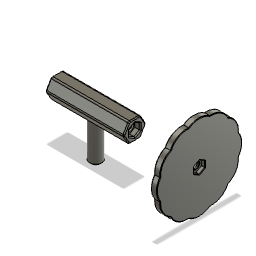
Interferometry Fine Adjust v5 (Autodesk Fusion 360 design; units mm, degrees)
Autodesk Fusion 360 part; units mm, degrees
note: some values were not read from the file. Chosen so that the rebuilt part matches the saved one: where a step starts; where a step ends.
sketch "Post" plane through (0, 0, 0) normal (0, 1, 0) x (1, 0, 0) in component "Fine Adjust Mount"
  circle A0 centre (0, 0) radius 6.25
  dimension "d1" = 12.5
  constraint coincident A0.centre origin
  measures "d1" diameter of A0
sketch "Shaft" plane through (0, 0, 0) normal (1, 0, 0) x (0, 0, -1) in component "Fine Adjust Mount"
  line L0 (0, 0) -> (5.5, 0) construction
  line L1 (0, 0) -> (0, -10) construction
  line L2 (5.5, 3.1754) -> (0, 6.3509)
  line L3 (0, 6.3509) -> (-5.5, 3.1754)
  line L4 (-5.5, 3.1754) -> (-5.5, -3.1754)
  line L5 (-5.5, -3.1754) -> (0, -6.3509)
  line L6 (0, -6.3509) -> (5.5, -3.1754)
  line L7 (5.5, -3.1754) -> (5.5, 3.1754)
  line L8 (5.7735, -10) -> (11.547, 0)
  line L9 (11.547, 0) -> (5.7735, 10)
  line L10 (5.7735, 10) -> (-5.7735, 10)
  line L11 (-5.7735, 10) -> (-11.547, 0)
  line L12 (-11.547, 0) -> (-5.7735, -10)
  line L13 (-5.7735, -10) -> (5.7735, -10)
  circle A0 centre (0, 0) radius 3.5
  dimension "d2" = 5.5
  dimension "d3" = 10
  dimension "d4" = 5.5
  dimension "d5" = 10
  dimension "d15" = 7
  constraint coincident L0.start L1.start
  constraint horizontal L0
  constraint perpendicular L0 L1
  constraint perpendicular L0 L7
  constraint perpendicular L1 L13
  measures "d2" distance of L0.start L0.end
  measures "d3" distance of L0.start L1.end
  measures "d4" distance of L0.start L7
  measures "d5" distance of L0.start L13
  measures "d15" diameter of A0
sketch "Disk" plane through (0, 0, 0) normal (1, 0, 0) x (0, 0, -1) in component "Fine Adjust Mount"
  line L0 (0, 0) -> (43.5, 0) construction
  line L1 (0, 0) -> (40.0859, 10.741) construction
  line L2 (0, 0) -> (42.5, 0) construction
  line L3 (0, 0) -> (40.0859, -10.741) construction
  line L4 (0, 0) -> (42.5, 0) construction
  arc A0 (40.0859, -10.741) -> (40.0859, 10.741) centre (24.8969, 0) ccw
  arc A1 (40.0859, 10.741) -> (29.3449, 29.3449) centre (21.5614, 12.4485) ccw
  arc A2 (29.3449, 29.3449) -> (10.741, 40.0859) centre (12.4485, 21.5614) ccw
  arc A3 (10.741, 40.0859) -> (-10.741, 40.0859) centre (0, 24.8969) ccw
  arc A4 (-10.741, 40.0859) -> (-29.3449, 29.3449) centre (-12.4485, 21.5614) ccw
  arc A5 (-29.3449, 29.3449) -> (-40.0859, 10.741) centre (-21.5614, 12.4485) ccw
  arc A6 (-40.0859, 10.741) -> (-40.0859, -10.741) centre (-24.8969, 0) ccw
  arc A7 (-40.0859, -10.741) -> (-29.3449, -29.3449) centre (-21.5614, -12.4485) ccw
  arc A8 (-29.3449, -29.3449) -> (-10.741, -40.0859) centre (-12.4485, -21.5614) ccw
  arc A9 (-10.741, -40.0859) -> (10.741, -40.0859) centre (0, -24.8969) ccw
  arc A10 (10.741, -40.0859) -> (29.3449, -29.3449) centre (12.4485, -21.5614) ccw
  arc A11 (29.3449, -29.3449) -> (40.0859, -10.741) centre (21.5614, -12.4485) ccw
  line L5 (5.5, 3.1754) -> (0, 6.3509)
  line L6 (0, 6.3509) -> (-5.5, 3.1754)
  line L7 (-5.5, 3.1754) -> (-5.5, -3.1754)
  line L8 (-5.5, -3.1754) -> (0, -6.3509)
  line L9 (0, -6.3509) -> (5.5, -3.1754)
  line L10 (5.5, -3.1754) -> (5.5, 3.1754)
  circle A12 centre (0, 0) radius 3.5
  dimension "d6" = 43.5
  dimension "d7" = 15
  dimension "d8" = 41.5
  dimension "d9" = 15
  dimension "d10" = 41.5
  dimension "d12" = 360
  dimension "d13" = 5.5
  dimension "d14" = 7
  constraint coincident L0.start L1.start
  constraint horizontal L0
  constraint horizontal L2
  constraint horizontal L4
  constraint coincident L0.end A0
  constraint perpendicular L4 L10
  measures "d6" distance of L0.start L0.end
  measures "d7" angle of L1 L2
  measures "d8" distance of L0.start L1.end
  measures "d9" angle of L3 L4
  measures "d10" distance of L0.start L3.end
  measures "d13" distance of L0.start L10
  measures "d14" diameter of A12
extrude "Extrude1" add sketch "Shaft" along normal mid plane 69 contours L2 L3 L4 L5 L6 L7 | L8 L9 L10 L11 L12 L13 makes body 1 in component "Fine Adjust Mount"
extrude "Extrude2" add sketch "Shaft" along normal mid plane 80 contours L8 L9 L10 L11 L12 L13 bodies 1 in component "Fine Adjust Mount"
extrude "Extrude3" add sketch "Post" along normal up to near side of body 1 and the other way blind 36 from surface at -11 bodies 1 in component "Fine Adjust Mount"
extrude "Extrude4" add sketch "Disk" along normal blind 6 separate body contours A0 A1 A2 A3 A4 A5 A6 A7 A8 A9 A10 A11 | L5 L6 L7 L8 L9 L10 makes body 2 in component "Fine Adjust Mount"
extrude "Extrude5" cut sketch "Disk" against normal blind 3.6667 from surface at 6 contours L5 L6 L7 L8 L9 L10 bodies 2 in component "Fine Adjust Mount"
move_body "Move1" bodies 2 to x (1, 0, 0) y (0, 1, 0) z (0, 0, 1) at (100, 0, 0) in component "Fine Adjust Mount"
fillet "Fillet2" radius 2 8 edges at (0, 10, 5.7735) (0, 10, -5.7735) (0, 0, -11.547) (0, 0, 11.547) (-21.1968, -10, 5.7735) (-21.1968, -10, -5.7735) (21.1968, -10, 5.7735) (21.1968, -10, -5.7735) on bodies 1 in component "Fine Adjust Mount"
chamfer "Chamfer2" [suppressed] in component "Fine Adjust Mount"
chamfer "Chamfer1" distance 1 angle 45 2 edges at (34.5, 1.2657, 3.2631) (-34.5, -1.2657, 3.2631) 2 faces at (-40, 0.3333, -7.3232) (40, 0.3333, -7.3232) on bodies 1 2 in component "Fine Adjust Mount"
chamfer "Chamfer1" distance 0.5 angle 45 2 edges at (102.3333, -1.2657, 3.2631) (100, 1.2657, 3.2631) 2 faces at (100, -13.8682, -24.1947) (106, 1.0585, -28.5573) on bodies 1 2 in component "Fine Adjust Mount"
chamfer "Chamfer1" distance 1 angle 45 1 edges at (-5.827, -47, -2.2601) on bodies 1 2 in component "Fine Adjust Mount"
component "Fine Adjust Mount" placed x (1, 0, 0) y (0, 1, 0) z (0, 0, 1) at (0, 0, 0)
equation "d1 = PostDiameter"
equation "d2 = NutApothem"
equation "d3 = ShaftApothem"
equation "d4 = d2"
equation "d5 = d3"
equation "d6 = DiskLD / 2"
equation "d7 = ( 360 / ( 2 * DiskLobes ) ) * 1 deg"
equation "d8 = ( DiskSD / 2 )"
equation "d9 = ( 360 / ( 2 * DiskLobes ) ) * 1 deg"
equation "d10 = ( DiskSD / 2 )"
equation "d13 = NutApothem"
equation "d14 = ClearanceHole"
equation "d15 = ClearanceHole"
equation "PostDiameter = 12.5 mm"
equation "NutApothem = 5.5 mm"
equation "ShaftApothem = 10 mm"
equation "DiskLD = 87 mm"
equation "DiskSD = 83 mm"
equation "DiskLobes = 12"
equation "ClearanceHole = 7 mm"
equation "PostLength = 37 mm"
equation "ShaftLength = 80 mm"
equation "DiskThickness = 6 mm"
equation "NutSeat = 5.5 mm"
equation "d27 = ShaftLength / 2 - NutSeat"
equation "d29 = ShaftLength / 2"
equation "d34 = PostLength - 1 mm"
equation "d36 = DiskThickness"
equation "d39 = -NutSeat / 1.5"
named bodies: "Post Mount", "Disk"
